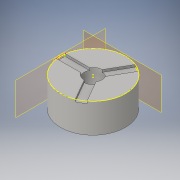
# Autodesk Inventor part: 3 jaww
Saved by Autodesk Inventor 2016 (Build 200138000, 138)
## iProperties
Created: 2017-06-20
Part Number: 3 jaww
Material: Generic
Document SubType Name: Modeling
Designer: M228854
Density: 1 g/cm^3
Appearance: Default
Author: M228854
Autodesk Inventor part; units mm, degrees
ref_plane "XZ Plane" through (0, 0, 0) normal (0, 1, 0) x (-1, 0, 0)
sketch "Sketch1" plane through (0, 0, 0) normal (0, 1, 0) x (-1, 0, 0)
  circle A0 centre (0, 0) radius 99.7
  constraints: 1 centre point, 1 coincident
extrude "Extrusion1" add sketch "Sketch1" along normal blind 90.9
sketch "Sketch2" plane through (0, 90.9, 0) normal (0, 1, 0) x (1, 0, 0)
  circle A0 centre (0, 0) radius 27.56
  dimension "d3" = 55.12
  constraints: 1 centre point, 1 coincident
  measures "d3" diameter of A0
extrude "Extrusion2" cut sketch "Sketch2" against normal blind 90.9
sketch "Sketch3" plane through (0, 90.9, 0) normal (0, 1, 0) x (1, 0, 0)
  circle A0 centre (0, 0) radius 99.7 projected
  line L0 (-99.7, 0) -> (-98.8062, 13.32)
  line L1 (-98.8062, 13.32) -> (-24.1274, 13.32)
  circle A1 centre (0, 0) radius 27.56 projected
  line L2 (-99.7, 0) -> (-98.8062, -13.32)
  line L3 (-98.8062, -13.32) -> (-24.1274, -13.32)
  line L4 (37.8676, -92.2287) -> (0.5282, -27.5549)
  line L5 (49.85, -86.3427) -> (37.8676, -92.2287)
  line L6 (49.85, -86.3427) -> (60.9386, -78.9087)
  line L7 (60.9386, -78.9087) -> (23.5992, -14.2349)
  line L8 (60.9386, 78.9087) -> (23.5992, 14.2349)
  line L9 (49.85, 86.3427) -> (60.9386, 78.9087)
  line L10 (49.85, 86.3427) -> (37.8676, 92.2287)
  line L11 (37.8676, 92.2287) -> (0.5282, 27.5549)
  line L12 (-24.1274, 13.32) -> (-24.1274, -13.32)
  line L13 (0.5282, 27.5549) -> (23.5992, 14.2349)
  line L14 (23.5992, -14.2349) -> (0.5282, -27.5549)
  dimension "d6" = 13.35
  dimension "d15" = 360
  constraints: 30 end point, 5 point on circle, 2 horizontal, 1 perpendicular, 1 vertical, 28 other
  measures "d6" distance of L0.start L0.end
ref_plane "Work Plane2" through (-99.7, 83.72, 0) normal (0.9978, 0, 0.067) x (0.067, 0, -0.9978)
sketch "Sketch4" plane through (-99.7, 83.72, 0) normal (0.9978, 0, 0.067) x (0.067, 0, -0.9978)
  line L0 (13.35, 0) -> (13.35, 7.18)
  line L1 (-13.2303, 7.18) -> (-13.2303, 0)
  point P0 (6.675, -83.72)
  constraints: 4 end point
ref_plane "Work Plane1" through (-98.8062, 83.72, 13.32) normal (0.9978, 0, -0.067) x (-0.067, 0, -0.9978)
sketch "Sketch5" plane through (-98.8062, 83.72, 13.32) normal (0.9978, 0, -0.067) x (-0.067, 0, -0.9978)
  line L0 (13.35, 0) -> (13.35, 7.18) projected
  line L1 (0, 0) -> (13.35, 0) projected
  line L2 (13.35, 5.7337) -> (13.35, 0)
  line L3 (13.35, 0) -> (0, 0)
  line L4 (0, 0) -> (0, 7.18)
  line L5 (0, 7.18) -> (0, 0) projected
  line L6 (106.375, 7.18) -> (-93.025, 7.18) projected
  point P0 (6.675, -83.72)
  point P1 (26.5803, 7.18)
  constraints: 6 end point, 2 collinear, 1 point on line, 1 vertical
extrude "Extrusion4" cut sketch "Sketch5" against normal blind 7.18
ref_plane "Work Plane3" through (-99.7, 83.72, 0) normal (0.9978, 0, 0.067) x (0.067, 0, -0.9978)
sketch "Sketch6" plane through (-99.7, 83.72, 0) normal (0.9978, 0, 0.067) x (0.067, 0, -0.9978)
  line L0 (0, 0) -> (13.35, 0) projected
  line L1 (0, 0) -> (0, 7.18) projected
  line L2 (0, 0) -> (0, 7.18)
  line L3 (13.35, 7.18) -> (18.3498, 7.18) projected
  line L4 (0, 7.18) -> (13.35, 7.18)
  line L5 (13.35, 0) -> (13.35, 7.18) projected
  line L6 (13.35, 7.18) -> (13.35, 0)
  line L7 (13.35, 0) -> (0, 0)
  point P0 (6.675, -83.72)
  constraints: 8 end point, 2 collinear, 2 perpendicular
extrude "Extrusion5" cut sketch "Sketch6" against normal blind 7.18
extrude "Extrusion6" cut sketch "Sketch3" against normal blind 7.18 contours L8 A1 L11 L10 L9 | L6 L5 L4 A1 L7 | L13 A1 | A1 L14 | L1 A1 L3 L2 L0
sketch "Sketch7" plane through (49.85, 83.72, -86.3427) normal (-0.5569, 0, 0.8306) x (0.8306, 0, 0.5569)
  line L0 (13.35, 7.18) -> (0, 7.18) projected
  line L1 (13.35, 0) -> (13.35, 7.18) projected
  line L2 (0, 7.18) -> (13.35, 7.18)
  line L3 (13.35, 0) -> (18.3498, 0) projected
  line L4 (13.35, 7.18) -> (13.35, 0)
  line L5 (0, 7.18) -> (0, 0) projected
  line L6 (13.35, 0) -> (0, 0)
  line L7 (0, 0) -> (0, 6.2119)
  line L8 (0, 7.18) -> (-13.2303, 7.18) projected
  line L9 (-13.2303, 4.6736) -> (0, 7.18)
  line L10 (0, 7.18) -> (0, 0)
  line L11 (-13.2303, -2.9965) -> (-13.2303, 4.6736)
  line L12 (-13.2303, 0) -> (-13.2303, 7.18) projected
  point P0 (6.675, -83.72)
  constraints: 14 end point, 3 perpendicular, 2 collinear, 1 point on line
extrude "Extrusion7" cut sketch "Sketch7" against normal blind 10 contours L1 L6 L5 L0
sketch "Sketch8" plane through (37.8676, 83.72, -92.2287) normal (-0.4409, 0, 0.8976) x (0.8976, 0, 0.4409)
  line L0 (0, 0) -> (0, 7.18) projected
  line L1 (-4.9998, 0) -> (0, 0) projected
  line L2 (0, 7.18) -> (0, 0)
  line L3 (0, 0) -> (13.35, 0) projected
  line L4 (0, 0) -> (13.35, 0)
  line L5 (13.35, 7.18) -> (13.35, 0) projected
  line L6 (13.35, 0) -> (13.35, 7.18)
  line L7 (0, 7.18) -> (13.35, 7.18) projected
  line L8 (13.35, 7.18) -> (0, 7.18)
  line L9 (0, 7.18) -> (0, 4.7035)
  point P0 (6.675, -83.72)
  constraints: 10 end point, 3 collinear, 1 point on line, 1 vertical
extrude "Extrusion8" cut sketch "Sketch8" against normal blind 10
sketch "Sketch10" plane through (49.85, 83.72, 86.3427) normal (-0.4409, 0, -0.8976) x (-0.8976, 0, 0.4409)
  line L0 (0, 7.18) -> (13.35, 7.18) projected
  line L1 (13.35, 7.18) -> (18.3498, 7.18) projected
  line L2 (0, 7.18) -> (13.35, 7.18)
  line L3 (13.35, 0) -> (18.3498, 0) projected
  line L4 (13.35, 7.18) -> (13.35, 0)
  line L5 (0, 0) -> (13.35, 0) projected
  line L6 (13.35, 0) -> (0, 0)
  line L7 (0, 0) -> (0, 7.18)
  line L8 (0, 7.18) -> (0, 0) projected
  point P0 (6.675, -83.72)
  constraints: 8 end point, 2 collinear, 1 horizontal, 1 perpendicular
extrude "Extrusion9" cut sketch "Sketch10" against normal blind 10
sketch "Sketch11" plane through (60.9386, 83.72, 78.9087) normal (-0.5569, 0, -0.8306) x (-0.8306, 0, 0.5569)
  line L0 (-4.9998, 7.18) -> (0, 7.18) projected
  line L1 (13.35, 7.18) -> (0, 7.18) projected
  line L2 (0, 7.18) -> (13.35, 7.18)
  line L3 (0, 0) -> (13.35, 0) projected
  line L4 (13.35, 7.18) -> (13.35, 0)
  line L5 (13.35, 0) -> (0, 0)
  line L6 (0, 0) -> (0, 7.18) projected
  line L7 (0, 0) -> (0, 7.18)
  point P0 (6.675, -83.72)
  constraints: 8 end point, 3 collinear, 1 perpendicular
extrude "Extrusion10" cut sketch "Sketch11" against normal blind 10
sketch "Sketch12" plane through (0, 90.9, 0) normal (0, 1, 0) x (1, 0, 0)
  arc A0 (37.8676, -92.2287) -> (60.9386, -78.9087) centre (0, 0) ccw projected
  arc A1 (-98.8062, -13.32) -> (37.8676, -92.2287) centre (0, 0) ccw projected
  arc A2 (-98.8062, 13.32) -> (-98.8062, -13.32) centre (0, 0) ccw projected
  arc A3 (37.8676, 92.2287) -> (-98.8062, 13.32) centre (0, 0) ccw projected
  arc A4 (60.9386, 78.9087) -> (37.8676, 92.2287) centre (0, 0) ccw projected
  arc A5 (60.9386, -78.9087) -> (60.9386, 78.9087) centre (0, 0) ccw projected
  circle A6 centre (0, 0) radius 99.7 projected
ref_plane "Work Plane5" through (-99.7, 0, 0) normal (1, 0, 0) x (0, 1, 0)
ref_plane "Work Plane6" through (0, 0, -99.7) normal (0, 0, 1) x (1, 0, 0)
sketch "Sketch13" plane through (0, 83.72, 0) normal (0, 1, 0) x (1, 0, 0)
  arc A0 (60.9386, 78.9087) -> (37.8676, 92.2287) centre (0, 0) ccw projected
sketch "Sketch14" plane through (-99.7, 83.72, 0) normal (0.9978, 0, 0.067) x (0.067, 0, -0.9978)
  point P0 (6.675, -83.72)
sketch "Sketch15" plane through (0, 0, 0) normal (0, -1, 0) x (1, 0, 0)
  circle A0 centre (0, 0) radius 27.56 projected
  circle A1 centre (19.78, 34.26) radius 10
  circle A2 centre (-39.56, 0) radius 10
  circle A3 centre (19.78, -34.26) radius 10
  point P0 (0.5282, 27.5549)
  point P1 (23.5992, 14.2349)
  dimension "d32" = 360
  constraints: 3 centre point, 2 coincident, 11 other
extrude "Extrusion11" cut sketch "Sketch15" against normal blind 40 contours A1 | A2 | A3
body "Solid1"
